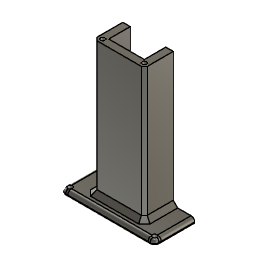
handlepiece2 (Autodesk Fusion 360 design; units mm, degrees)
Autodesk Fusion 360 part; units mm, degrees
sketch "Sketch1" plane through (0, 0, 0) normal (0, 0, 1) x (1, 0, 0)
  line L0 (-28.5, -24) -> (-28.5, 24)
  line L1 (-28.5, 24) -> (28.5, 24)
  line L2 (28.5, 24) -> (28.5, -24)
  line L3 (-28.5, -24) -> (28.5, -24)
  circle A0 centre (-28.5, 24) radius 1.5
  circle A1 centre (28.5, 24) radius 1.5
  circle A2 centre (-28.5, -24) radius 1.5
  circle A3 centre (28.5, -24) radius 1.5
  line L4 (0, 24) -> (0, -24)
  line L5 (0, 0) -> (-28.5, 0)
  line L6 (-31.5, -27) -> (31.5, -27)
  line L7 (31.5, 27) -> (31.5, -27)
  line L8 (-31.5, 27) -> (31.5, 27)
  line L9 (-31.5, -27) -> (-31.5, 27)
  dimension "d1" = 3
  dimension "d2" = 3
  dimension "d3" = 3
  dimension "d4" = 3
  dimension "d5" = -3
  constraint perpendicular L0 L3
  constraint coincident L0.end L1.start
  constraint coincident L1.end L2.start
  constraint coincident L0.start L3.start
  constraint coincident L2.end L3.end
  constraint midpoint L1 L4.start
  constraint midpoint L3 L4.end
  constraint midpoint L4 L5.start
  constraint midpoint L0 L5.end
  constraint perpendicular L0 L5
  measures "d1" diameter of A0
  measures "d2" diameter of A1
  measures "d3" diameter of A2
  measures "d4" diameter of A3
extrude "Extrude1" add sketch "Sketch1" along normal blind 3 contours L0 L3 A2 L4 L5 | L0 L1 A0 L4 L5 | L1 L2 L3 A1 A3 L4 | L6 L7 L8 L9
sketch "Sketch2" plane through (0, 0, 3) normal (0, 0, 1) x (-1, 0, 0)
  circle A0 centre (-28.5, -24) radius 1.5
  circle A1 centre (28.5, 24) radius 1.5
  circle A2 centre (28.5, -24) radius 1.5
  circle A3 centre (-28.5, 24) radius 1.5
  line L0 (31.5, 27) -> (-31.5, 27)
  line L1 (-31.5, 27) -> (-31.5, -27)
  line L2 (-31.5, -27) -> (31.5, -27)
  line L3 (31.5, -27) -> (31.5, 27)
  line L4 (-15, -19.5) -> (15, -19.5)
  line L5 (12, -14.5) -> (-12, -14.5)
  circle A4 centre (14, -16.5) radius 1.5
  line L6 (15, -19.5) -> (17, -17.5)
  line L7 (17, -17.5) -> (17, 0)
  line L8 (17, 0) -> (12, 0)
  line L9 (12, 0) -> (12, -14.5)
  line L10 (-12, -14.5) -> (-12, 0)
  line L11 (-12, 0) -> (-17, 0)
  line L12 (-17, 0) -> (-17, -17.5)
  line L13 (-17, -17.5) -> (-15, -19.5)
  circle A5 centre (-14, -16.5) radius 1.5
  line L14 (12, 0) -> (-12, 0)
  line L15 (0, 0) -> (0, -7.25)
  line L16 (12, 0) -> (12, 14.5)
  line L17 (17, 17.5) -> (17, 0)
  line L18 (17, 0) -> (12, 0)
  line L19 (-15, 19.5) -> (15, 19.5)
  line L20 (12, 14.5) -> (-12, 14.5)
  line L21 (-12, 14.5) -> (-12, 0)
  circle A6 centre (14, 16.5) radius 1.5
  circle A7 centre (-14, 16.5) radius 1.5
  line L22 (-17, 17.5) -> (-15, 19.5)
  line L23 (-17, 0) -> (-17, 17.5)
  line L24 (-12, 0) -> (-17, 0)
  line L25 (15, 19.5) -> (17, 17.5)
  constraint perpendicular L10 L14
  constraint midpoint L14 L15.start
  constraint perpendicular L14 L15
  constraint symmetric L12.end L14 L22.start
  constraint symmetric L4.start L14 L19.start
  constraint symmetric L4.end L14 L19.end
  constraint symmetric L6.end L14 L17.start
  constraint symmetric L8.end L14 L9.start
  constraint symmetric L5.start L14 L16.end
  constraint symmetric L5.end L14 L20.end
  constraint symmetric L10.end L14 L11.start
  constraint symmetric L11.end L14 L12.start
  constraint symmetric L7.end L14 L8.start
  constraint symmetric A4 L14 A6
  constraint symmetric A5 L14 A7
extrude "Extrude2" add sketch "Sketch2" along normal blind 90 contours L4 L5 L6 L7 L8 L9 L10 L11 L12 L13 L18 L24 | L8 L11 L16 L17 L18 L19 L20 L21 L22 L23 L24 L25
fillet "Fillet1" radius 3 4 edges at (-31.5, -27, 1.5) (31.5, -27, 1.5) (31.5, 27, 1.5) (-31.5, 27, 1.5)
fillet "Fillet2" radius 2.5 8 edges at (30.6213, 26.1213, 3) (0, 27, 3) (-30.6213, 26.1213, 3) (-31.5, 0, 3) (-30.6213, -26.1213, 3) (0, -27, 3) (30.6213, -26.1213, 3) (31.5, 0, 3)
chamfer "Chamfer1" distance 3 angle 45 8 edges at (0, 19.5, 3) (17, 0, 3) (16, 18.5, 3) (-16, 18.5, 3) (-16, -18.5, 3) (-17, 0, 3) (0, -19.5, 3) (16, -18.5, 3)
sketch "Sketch3" plane through (0, 19.5, 0) normal (0, 1, 0) x (-1, 0, 0)
  line L0 (15, 6) -> (15, 93)
  line L1 (15, 93) -> (-15, 93)
  line L2 (-15, 93) -> (-15, 6)
  line L3 (-15, 49.5) -> (15, 49.5)
  circle A0 centre (0, 49.5) radius 9.5
  line L4 (-15, 6) -> (15, 6)
  dimension "d12" = 19
  constraint midpoint L2 L3.start
  constraint midpoint L0 L3.end
  constraint midpoint L3 A0.centre
  measures "d12" diameter of A0
extrude "Extrude3" cut sketch "Sketch3" against normal blind 6 contours L3 A0 | L3 A0
sketch "Sketch4" plane through (0, 0, 93) normal (0, 0, 1) x (-1, 0, 0)
  circle A0 centre (14, -16.5) radius 1.5
  circle A1 centre (14, 16.5) radius 1.5
  circle A2 centre (-14, -16.5) radius 1.5
  line L0 (12, 14.5) -> (12, -14.5)
  line L1 (12, -14.5) -> (-12, -14.5)
  line L2 (-12, -14.5) -> (-12, 14.5)
  line L3 (-12, 14.5) -> (12, 14.5)
  circle A3 centre (-14, 16.5) radius 1.5
  line L4 (-17, 17.5) -> (-17, -17.5)
  line L5 (-17, -17.5) -> (-15, -19.5)
  line L6 (-15, -19.5) -> (15, -19.5)
  line L7 (15, -19.5) -> (17, -17.5)
  line L8 (17, -17.5) -> (17, 17.5)
  line L9 (17, 17.5) -> (15, 19.5)
  line L10 (15, 19.5) -> (-15, 19.5)
  line L11 (-15, 19.5) -> (-17, 17.5)
  line L12 (-50, 0) -> (50, 0)
  line L13 (50, 0) -> (33.9234, 54.6299)
  line L14 (33.9234, 54.6299) -> (-46.2592, 44.9375)
  line L15 (-46.2592, 44.9375) -> (-50, 0)
  line L16 (12, 14.5) -> (-12, 14.5)
  line L17 (-12, 14.5) -> (-12, -14.5)
  line L18 (-12, -14.5) -> (12, -14.5)
  line L19 (12, -14.5) -> (12, 14.5)
  line L20 (-50, 0) -> (-64.2202, -68.1179)
  line L21 (-64.2202, -68.1179) -> (43.9074, -45.7813)
  line L22 (43.9074, -45.7813) -> (50, 0)
  constraint horizontal L12
extrude "Extrude4" cut sketch "Sketch4" against normal blind 500 contours A0 | A2 | L0 L2 L3 L12 L16 L17 L19 | L0 L1 L2 L4 L5 L6 L7 L8 L12 L17 L18 L19 | L0 L1 L2 L12 L17 L18 L19 | L4 L5 L6 L7 L8 L12 L20 L21 L22
